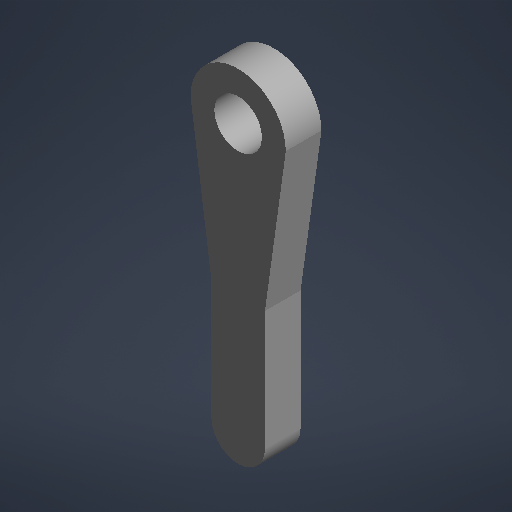
# Autodesk Inventor part: drop_arm
Saved by Autodesk Inventor 2026 (Build 300175050, 175E)
## iProperties
Part Number: drop_arm
Material: Generic
Document SubType Name: Modeling
Designer: Administrator
Appearance: Default
Author: Administrator
Autodesk Inventor part; units mm, degrees
ref_plane "YZ Plane" through (0, 0, 0) normal (1, 0, 0) x (0, 1, 0)
ref_plane "XZ Plane" through (0, 0, 0) normal (0, 1, 0) x (-1, 0, 0)
ref_plane "XY Plane" through (0, 0, 0) normal (0, 0, 1) x (1, 0, 0)
sketch "Sketch1" plane through (0, 0, 0) normal (0, 0, 1) x (1, 0, 0)
  line L0 (-45, 0) -> (-45, 200)
  line L1 (-45, 200) -> (-80, 450)
  arc A0 (80, 450) -> (-80, 450) centre (0, 450) ccw
  line L2 (80, 450) -> (45, 200)
  line L3 (45, 200) -> (45, 0)
  arc A1 (-45, 0) -> (45, 0) centre (0, 0) ccw
  constraints: 8 end point, 4 point on circle, 2 centre point
extrude "Extrusion1" add sketch "Sketch1" along normal blind 60
sketch "Sketch2" plane through (0, 0, 0) normal (0, 0, 1) x (1, 0, 0)
  circle A0 centre (0, 450) radius 40
  constraints: 1 centre point
extrude "Extrusion2" add sketch "Sketch2" along normal blind 60 separate body
combine bodies "Combine1" operation type subtract main body 1 bodies to subtract 2
body "Solid1"
